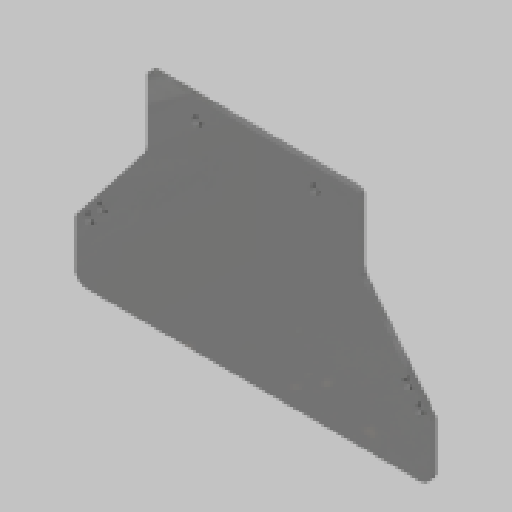
# Autodesk Inventor part: PolyRamp1
Saved by Autodesk Inventor 2026.1 (Build 301233000, 233)
## iProperties
Created: 2025-09-08
Part Number: PolyRamp1
Material: Polycarbonate, Smoke
Document SubType Name: Modeling
Designer: Teddy
Density: 1.2 g/cm^3
Appearance: Polycarbonate - Smoked
Author: Teddy
Autodesk Inventor part; units mm, degrees
ref_plane "YZ Plane" through (0, 0, 0) normal (1, 0, 0) x (0, 1, 0)
ref_plane "XZ Plane" through (0, 0, 0) normal (0, 1, 0) x (-1, 0, 0)
ref_plane "XY Plane" through (0, 0, 0) normal (0, 0, 1) x (1, 0, 0)
ref_plane "Work Plane1" through (34.6079, -50.31, 0) normal (0, 0, 1) x (1, 0, 0)
sketch "Sketch1" plane through (34.6079, -50.31, 0) normal (0, 0, 1) x (1, 0, 0)
  circle A0 centre (-188.0909, 15.5737) radius 4.445
  circle A1 centre (-194.7256, 7.071) radius 4.445
  circle A2 centre (-23.7989, 15.7359) radius 4.445
  circle A3 centre (-17.1643, 7.2332) radius 4.445
  line L0 (-188.0953, 20.0187) -> (-23.8033, 20.1809) construction
  line L1 (-48.7316, 54.9146) -> (8.842, -18.8701)
  line L2 (-17.1602, 2.7882) -> (-194.7215, 2.626) construction
  line L3 (-163.0316, 54.9146) -> (-220.6053, -18.8701)
  line L4 (-174.2634, 54.9146) -> (-39.5431, 54.9146) construction
  line L5 (-163.0316, 54.9146) -> (-163.0316, 93.0146)
  line L6 (-163.0316, 93.0146) -> (-48.7316, 93.0146)
  line L7 (-48.7316, 93.0146) -> (-48.7316, 54.9146)
  line L8 (-286.9371, -18.8701) -> (2.6787, -18.8701)
  line L9 (-201.5553, 5.5438) -> (-201.5553, -18.8701)
  line L10 (-10.208, 5.5438) -> (-10.208, -18.8701)
  line L11 (-201.5553, -18.8701) -> (-201.5553, -25.2201)
  line L12 (-201.5553, -25.2201) -> (-10.208, -25.2201)
  line L13 (-10.208, -25.2201) -> (-10.208, -18.8701)
  circle A4 centre (-194.7256, 7.071) radius 2.286 projected
  circle A5 centre (-188.0909, 15.5737) radius 2.286 projected
  circle A6 centre (-23.7989, 15.7359) radius 2.286 projected
  circle A7 centre (-17.1643, 7.2332) radius 2.286 projected
  circle A8 centre (-137.0599, 81.1641) radius 2.286 projected
  circle A9 centre (-73.5599, 81.1641) radius 2.286 projected
  point P0 (-34.6079, 50.31)
  point P1 (-20.2945, 18.4704)
  point P2 (-13.6599, 9.9676)
  point P3 (-191.5953, 18.3082)
  point P4 (-198.23, 9.8054)
  dimension "d0" = 8.89
  dimension "d1" = 8.89
  dimension "d2" = 8.89
  dimension "d3" = 8.89
  dimension "d6" = 114.3
  dimension "d7" = 38.1
  dimension "d10" = 19.05
  dimension "d11" = 19.05
  dimension "d12" = 6.35
  constraints: 28 end point, 12 point on line, 8 point on circle, 8 tangent, 6 perpendicular, 4 centre point, 4 coincident, 2 horizontal, 2 vertical
  measures "d0" diameter of A0
  measures "d1" diameter of A1
  measures "d2" diameter of A2
  measures "d3" diameter of A3
  measures "d6" distance of L5.end L6.end
  measures "d7" distance of L3.start L5.end
  measures "d10" distance from line of L1.end L10
  measures "d11" distance from line of L3.end L9
  measures "d12" distance between parallel lines of L8 L12
extrude "Extrusion1" add sketch "Sketch1" along normal blind 3.175 contours A0 | A1 | A3 | A2 | L3 L5 L6 L7 L1 L10 L8 L9 | L8 L13 L12 L11
fillet "Fillet1" radius 3.175 4 edges at (-128.4238, 42.7045, 1.5875) (-14.1238, 42.7045, 1.5875) (-166.9474, -44.7663, 1.5875) (24.3999, -44.7663, 1.5875)
fillet "Fillet2" radius 6.35 2 edges at (-128.4238, 4.6045, 1.5875) (-14.1238, 4.6045, 1.5875)
fillet "Fillet3" radius 6.35 2 edges at (24.3999, -75.5302, 1.5875) (-166.9474, -75.5302, 1.5875)
body "Solid1"
